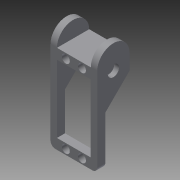
# Autodesk Inventor part: new_shoulder_modified
Saved by Autodesk Inventor 2014 SP1 (Build 180222100, 222)
## iProperties
Created: 2014-12-06
Part Number: new_shoulder_modified
Material: Générique
Document SubType Name: Modeling
Designer: astralien3000
Density: 1 g/cm^3
Appearance: Par défaut
d1: 6,400 mm
d2: 21,000 mm
d3: 4,000 mm
d4: 4,000 mm
d5: 10,500 mm
d6: 42,000 mm
d7: 10,000 mm
d8: 35,541 mm
d9: 6,400 mm
d10: 20,000 mm
d11: 0,00 deg
d12: 50,000 mm
d13: 7,000 mm
d14: 3,000 mm
d15: 0,00 deg
d16: 50,000 mm
d17: 7,000 mm
d18: 3,000 mm
d19: 0,00 deg
d30: 6,400 mm
d31: 19,800 mm
d32: 9,900 mm
d33: 5,000 mm
d34: 5,000 mm
d35: 5,000 mm
d36: 5,000 mm
d37: 3,200 mm
d38: 3,200 mm
d40: 0,00 deg
d41: 30,000 mm
d42: 15,000 mm
d43: 0,00 deg
d44: 15,000 mm
d47: 3,000 mm
d48: 10,000 mm
d29: 6,400 mm
Author: astralien3000
Autodesk Inventor part; units mm, degrees
ref_plane "YZ Plane" through (0, 0, 0) normal (1, 0, 0) x (0, 1, 0)
ref_plane "XZ Plane" through (0, 0, 0) normal (0, 1, 0) x (-1, 0, 0)
ref_plane "XY Plane" through (0, 0, 0) normal (0, 0, 1) x (1, 0, 0)
sketch "Esquisse1" plane through (0, 0, 0) normal (0, 1, 0) x (-1, 0, 0)
  line L0 (-14.5, 51.941) -> (-10.5, 51.941)
  line L1 (-10.5, 51.941) -> (-10.5, -12.859)
  line L2 (-10.5, -12.859) -> (-14.5, -12.859)
  line L3 (-14.5, -12.859) -> (-14.5, 51.941)
  line L4 (10.5, 51.941) -> (14.5, 51.941)
  line L5 (14.5, 51.941) -> (14.5, -12.859)
  line L6 (14.5, -12.859) -> (10.5, -12.859)
  line L7 (10.5, -12.859) -> (10.5, 51.941)
  line L8 (-10.5, -6.459) -> (10.5, -6.459)
  line L9 (10.5, -6.459) -> (10.5, -12.859)
  line L10 (10.5, -12.859) -> (-10.5, -12.859)
  line L11 (-10.5, -12.859) -> (-10.5, -6.459)
  line L12 (-10.5, 41.941) -> (10.5, 41.941)
  line L13 (10.5, 41.941) -> (10.5, 35.541)
  line L14 (10.5, 35.541) -> (-10.5, 35.541)
  line L15 (-10.5, 35.541) -> (-10.5, 41.941)
  line L16 (10.5, -12.859) -> (14.5, -12.859)
  point P0 (0, 0)
  dimension "d1" = 6.4
  dimension "d2" = 21
  dimension "d3" = 4
  dimension "d4" = 4
  dimension "d5" = 10.5
  dimension "d6" = 42
  dimension "d7" = 10
  dimension "d8" = 35.541
  dimension "d9" = 6.4
  constraints: 34 end point, 9 equal length, 4 horizontal, 4 perpendicular, 4 point on line, 3 collinear
  measures "d1" distance between parallel lines of L14 L12
  measures "d2" distance between parallel lines of L1 L7
  measures "d3" distance between parallel lines of L7 L5
  measures "d4" distance between parallel lines of L3 L1
  measures "d5" distance from line of point (0, 0) L7
  measures "d6" distance between parallel lines of L8 L14
  measures "d7" distance between parallel lines of L4 L12
  measures "d8" distance from line of point (0, 0) L14
  measures "d9" distance between parallel lines of L16 L8
extrude "Extrusion1" add sketch "Esquisse1" along normal blind 20 contours L0 L1 L2 L3 | L12 L7 L14 L1 | L1 L8 L7 L10 | L7 L4 L5 L6
sketch "Esquisse2" plane through (14.5, 0, 51.941) normal (1, 0, 0) x (0, 0, -1)
  line L0 (64.8, 0) -> (64.8, 20) projected
  line L1 (0, 0) -> (0, 20) projected
  line L2 (0, 10) -> (64.8, 10) construction
  circle A0 centre (14.8, 10) radius 3.5
  point P0 (51.941, 0)
  dimension "d12" = 50
  dimension "d13" = 7
  constraints: 2 end point, 2 midpoint, 1 centre point, 1 point on line
  measures "d12" distance from line of A0.centre L0
  measures "d13" diameter of A0
extrude "Extrusion2" cut sketch "Esquisse2" against normal blind 3
sketch "Esquisse3" plane through (-14.5, 0, -12.859) normal (-1, 0, 0) x (0, 0, 1)
  line L0 (64.8, 0) -> (64.8, 20) projected
  line L1 (0, 0) -> (0, 20) projected
  line L2 (64.8, 10) -> (0, 10) construction
  circle A0 centre (50, 10) radius 3.5
  point P0 (12.859, 0)
  dimension "d16" = 50
  dimension "d17" = 7
  constraints: 2 end point, 2 midpoint, 1 centre point, 1 point on line
  measures "d16" distance from line of L1 A0.centre
  measures "d17" diameter of A0
extrude "Extrusion3" cut sketch "Esquisse3" against normal blind 3
sketch "Esquisse5" plane through (0, 20, 0) normal (0, 1, 0) x (1, 0, 0)
  line L0 (10.5, -35.541) -> (-10.5, -35.541) projected
  line L1 (14.5, 12.859) -> (-14.5, 12.859) projected
  line L2 (-10.5, -41.941) -> (10.5, -41.941) projected
  line L3 (-9.9, 12.859) -> (9.9, 12.859)
  line L4 (9.9, 12.859) -> (9.9, 6.459)
  line L5 (9.9, 6.459) -> (-9.9, 6.459)
  line L6 (-9.9, 6.459) -> (-9.9, 12.859)
  line L7 (-9.9, -41.941) -> (9.9, -41.941)
  line L8 (9.9, -41.941) -> (9.9, -35.541)
  line L9 (9.9, -35.541) -> (-9.9, -35.541)
  line L10 (-9.9, -35.541) -> (-9.9, -41.941)
  line L11 (0, 12.859) -> (0, -41.941)
  circle A0 centre (5, 9.659) radius 2.5
  circle A1 centre (5, -38.741) radius 2.5
  circle A2 centre (-5, 9.659) radius 2.5
  circle A3 centre (-5, -38.741) radius 2.5
  point P0 (0, 0)
  dimension "d29" = 6.4
  dimension "d30" = 6.4
  dimension "d31" = 19.8
  dimension "d32" = 9.9
  dimension "d33" = 5
  dimension "d34" = 5
  dimension "d35" = 5
  dimension "d36" = 5
  dimension "d37" = 3.2
  dimension "d38" = 3.2
  constraints: 18 end point, 4 centre point, 4 parallel, 3 point on line, 2 collinear, 2 horizontal, 2 midpoint, 2 perpendicular, 2 symmetric about line, 2 other
  measures "d29" distance between parallel lines of L7 L9
  measures "d30" distance between parallel lines of L1 L5
  measures "d31" distance between parallel lines of L4 L6
  measures "d32" distance from line of point (0, 0) L4
  measures "d33" diameter of A0
  measures "d34" diameter of A1
  measures "d35" distance from line of L11 A0.centre
  measures "d36" distance from line of L11 A1.centre
  measures "d37" distance from line of L2 A1.centre
  measures "d38" distance from line of L1 A0.centre
extrude "Extrusion5" cut sketch "Esquisse5" against normal through all contours A0 | A1 | A2 | A3
sketch "Esquisse6" plane through (0, 20, 0) normal (0, 1, 0) x (1, 0, 0)
  circle A0 centre (-5, 9.659) radius 2.5 projected
  circle A1 centre (5, 9.659) radius 2.5 projected
  line L0 (14.5, -51.941) -> (14.5, 12.859) projected
  line L1 (-14.5, 12.859) -> (14.5, 12.859)
  line L2 (14.5, 12.859) -> (14.5, -17.141)
  line L3 (14.5, -17.141) -> (-14.5, -17.141)
  line L4 (-14.5, -17.141) -> (-14.5, 12.859)
  point P0 (0, 0)
  dimension "d41" = 30
  constraints: 8 end point, 2 parallel, 1 horizontal, 1 perpendicular, 1 point on line
  measures "d41" distance between parallel lines of L1 L3
extrude "Extrusion6" cut sketch "Esquisse6" against normal blind 15
chamfer "Chanfrein1" distance 15 angle 45 2 edges at (12.5, 20, 17.141) (-12.5, 20, 17.141)
fillet "Congé1" radius 3 2 edges at (-14.5, 2.5, -12.859) (14.5, 2.5, -12.859)
fillet "Congé2" radius 10 4 edges at (-12.5, 0, 51.941) (12.5, 0, 51.941) (-12.5, 20, 51.941) (12.5, 20, 51.941)
equation "\"d4\" = d3"
equation "\"d5\" = 0.5 * d2"
equation "\"d9\" = d1"
equation "\"d30\" = d29"
equation "\"d32\" = 0.5 * d31"
equation "\"d34\" = d33"
equation "\"d38\" = d37"
